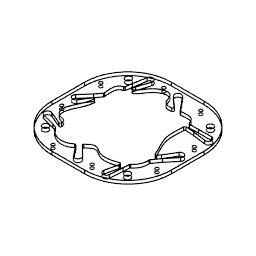
MidPlateShell_v29 (Autodesk Fusion 360 design; units mm, degrees)
Autodesk Fusion 360 part; units mm, degrees
(part 1 of 2)
sketch "Sketch1" plane through (0, 0, 0) normal (0, 0, 1) x (1, 0, 0)
  line L0 (-33.4, -17.4) -> (-33.4, 33.4) construction
  line L1 (-33.4, 33.4) -> (-27.4, 33.4) construction
  line L2 (-33.4, -17.4) -> (-36.4, -17.4)
  line L3 (-36.4, -17.4) -> (-36.4, -27.4)
  line L4 (-36.4, -27.4) -> (-33.4, -27.4)
  line L5 (-33.4, -27.4) -> (-33.4, -17.4)
  line L6 (-27.4, 33.4) -> (-17.4, 33.4)
  line L7 (-17.4, 33.4) -> (-17.4, 36.4)
  line L8 (-17.4, 36.4) -> (-27.4, 36.4)
  line L9 (-27.4, 36.4) -> (-27.4, 33.4)
  line L10 (-17.4, 33.4) -> (33.4, 33.4) construction
  line L11 (33.4, 33.4) -> (33.4, 27.4) construction
  line L12 (33.4, 27.4) -> (36.4, 27.4)
  line L13 (36.4, 27.4) -> (36.4, 17.4)
  line L14 (36.4, 17.4) -> (33.4, 17.4)
  line L15 (33.4, 17.4) -> (33.4, 27.4)
  line L16 (33.4, 17.4) -> (33.4, -33.4) construction
  line L17 (33.4, -33.4) -> (27.4, -33.4) construction
  line L18 (27.4, -33.4) -> (17.4, -33.4)
  line L19 (17.4, -33.4) -> (17.4, -36.4)
  line L20 (17.4, -36.4) -> (27.4, -36.4)
  line L21 (27.4, -36.4) -> (27.4, -33.4)
  line L22 (17.4, -33.4) -> (-33.4, -33.4) construction
  line L23 (-33.4, -33.4) -> (-33.4, -27.4) construction
  line L24 (33.4, 33.4) -> (-33.4, -33.4) construction
  line L25 (33.4, -33.4) -> (-33.4, 33.4) construction
  line L26 (55, -55) -> (-55, -55)
  line L27 (-55, -55) -> (-55, 55)
  line L28 (-55, 55) -> (55, 55)
  line L29 (55, 55) -> (55, -55)
  line L30 (55, -55) -> (-55, 55) construction
  line L31 (-55, -55) -> (55, 55) construction
  line L32 (-34.9, -17.4) -> (-34.9, -7.75) construction
  line L33 (-34.9, -7.75) -> (-38.15, -7.75) construction
  circle A0 centre (-38.15, -7.75) radius 1.25
  line L34 (-34.9, -27.4) -> (-34.9, -38.15) construction
  line L35 (-34.9, -38.15) -> (-37.75, -38.15) construction
  circle A1 centre (-37.75, -38.15) radius 1.25
  circle A2 centre (38.15, -37.75) radius 1.25
  circle A3 centre (7.75, -38.15) radius 1.25
  circle A4 centre (37.75, 38.15) radius 1.25
  circle A5 centre (38.15, 7.75) radius 1.25
  circle A6 centre (-38.15, 37.75) radius 1.25
  circle A7 centre (-7.75, 38.15) radius 1.25
  constraint vertical L0
  constraint perpendicular L0 L1
  constraint horizontal L2
  constraint vertical L3
  constraint horizontal L4
  constraint vertical L5
  constraint horizontal L6
  constraint vertical L7
  constraint horizontal L8
  constraint vertical L9
  constraint perpendicular L7 L10
  constraint perpendicular L10 L11
  constraint horizontal L12
  constraint vertical L13
  constraint horizontal L14
  constraint vertical L15
  constraint perpendicular L14 L16
  constraint perpendicular L16 L17
  constraint horizontal L18
  constraint vertical L19
  constraint horizontal L20
  constraint vertical L21
  constraint perpendicular L19 L22
  constraint coincident origin L24
  constraint coincident origin L25
  constraint horizontal L26
  constraint perpendicular L26 L27
  constraint parallel L26 L28
  constraint parallel L27 L29
  constraint coincident L30 origin
  constraint coincident L31 origin
  constraint midpoint L2 L32.start
  constraint perpendicular L2 L32
  constraint perpendicular L32 L33
  constraint coincident L33.end A0.centre
  constraint midpoint L4 L34.start
  constraint perpendicular L4 L34
  constraint perpendicular L34 L35
  constraint coincident L35.end A1.centre
  measures "d1" distance of L0.start L0.end
  measures "d2" distance of L0.end L1.end
  measures "d3" distance of L0.start L2.end
  measures "d4" distance of L0.start L4.end
  measures "d5" distance of L1.end L6.end
  measures "d6" distance of L1.end L8.end
  measures "d7" distance of L6.end L10.end
  measures "d8" distance of L10.end L11.end
  measures "d9" distance of L11.end L12.end
  measures "d10" distance of L11.end L14.end
  measures "d11" distance of L14.end L16.end
  measures "d12" distance of L16.end L17.end
  measures "d13" distance of L17.end L18.end
  measures "d14" distance of L17.end L20.end
  measures "d15" distance of L18.end L22.end
  measures "d16" distance of L27.end L28.end
  measures "d17" distance of L26.end L27.end
  measures "d22" distance of L32.start L32.end
  measures "d23" distance of L32.end L33.end
  measures "d24" diameter of A0
  measures "d25" distance of L34.start L34.end
  measures "d26" distance of L34.end L35.end
  measures "d27" diameter of A1
extrude "Extrude1" add sketch "Sketch1" along normal blind 3 contours L2 L3 L4 L5 | L6 L7 L8 L9 | L12 L13 L14 L15 | L18 L19 L20 L21 | L26 L27 L28 L29 | A0 | A1 | A2 | A3 | A4 | A5 | A6 | A7 picked at (-35.4, -24.066667) picked at (-24.066667, 35.4) picked at (34.4, 24.066667) picked at (20.733333, -34.4) picked at (-5.8, 11.133333) picked at (-38.302225, -8.262066) picked at (-38.630134, -38.247182) picked at (37.269866, -37.847182) picked at (7.417812, -38.501562) picked at (36.869866, 38.052818) picked at (37.997775, 7.237934) picked at (-39.030134, 37.652818) picked at (-8.082188, 37.798438)
fillet "Fillet1" radius 40 4 edges at (-55, 55, 1.5) (55, 55, 1.5) (55, -55, 1.5) (-55, -55, 1.5)
other "Sketch1 (1)"
sketch "sketch 2514" plane through (0, 0, 0) normal (0, 0, 1) x (1, 0, 0)
  line L0 (55, -55) -> (-55, -55)
  line L1 (-55, -55) -> (-55, 55)
  line L2 (-55, 55) -> (55, 55)
  line L3 (55, 55) -> (55, -55)
  circle A0 centre (-27, 47.000001) radius 3
  circle A1 centre (-1, 47.000001) radius 3
  circle A2 centre (-47.000001, -1) radius 3
  circle A3 centre (-47.000001, -27) radius 3
  circle A4 centre (3.826834, 9.238795) radius 2.1
  line L4 (3.826834, 9.238795) -> (0, 0) construction
  circle A5 centre (-3.826834, 9.238795) radius 2.1
  circle A6 centre (-9.238795, 3.826834) radius 2.1
  circle A7 centre (-9.238795, -3.826834) radius 2.1
  circle A8 centre (-3.826834, -9.238795) radius 2.1
  circle A9 centre (3.826834, -9.238795) radius 2.1
  circle A10 centre (9.238795, -3.826834) radius 2.1
  circle A11 centre (9.238795, 3.826834) radius 2.1
  circle A12 centre (-47.000001, -27) radius 3
  circle A13 centre (-47.000001, -1) radius 3
  circle A14 centre (27, -47.000001) radius 3
  circle A15 centre (1, -47.000001) radius 3
  circle A16 centre (47.000001, 27) radius 3
  circle A17 centre (47.000001, 1) radius 3
  line L5 (3.826834, 9.238795) -> (-7.355951, 51.448425) construction
  line L6 (-3.826709, 9.238713) -> (-39.148117, 32.338774) construction
  line L7 (-9.224092, 3.83023) -> (-38.107832, -2.83954) construction
  line L8 (-9.238692, -3.826753) -> (-45.731263, -32.409069) construction
  line L9 (-3.841818, -9.257167) -> (-24.537186, -34.631992) construction
  line L10 (3.826834, -9.238795) -> (20.713135, -35.705512) construction
  line L11 (9.238772, -3.82683) -> (32.789694, -8.144866) construction
  line L12 (9.238795, 3.826834) -> (22.419532, 22.467528) construction
  line L13 (0, 0) -> (0, 3) construction
  line L14 (-38.107832, -2.83954) -> (1, -47.000001) construction
  line L15 (32.789694, -8.144866) -> (27, -47.000001) construction
  line L16 (20.713135, -35.705512) -> (47.000001, 1) construction
  line L17 (-39.148117, 32.338774) -> (47.000001, 27) construction
  line L18 (22.419532, 22.467528) -> (-1, 47.000001) construction
  line L19 (-45.731263, -32.409069) -> (-27, 47.000001) construction
  line L20 (-24.537186, -34.631992) -> (-47.000001, -27) construction
  line L21 (-7.355951, 51.448425) -> (-47.000001, -1) construction
  circle A18 centre (-26.92648, -6.415459) radius 6 construction
  circle A19 centre (-26.552885, -27.610279) radius 6 construction
  circle A20 centre (21, -25) radius 6 construction
  circle A21 centre (26, -13) radius 6 construction
  circle A22 centre (14.668303, 21.897871) radius 6 construction
  circle A23 centre (-10, 38.000001) radius 6 construction
  circle A24 centre (-16.884287, 24.947529) radius 6 construction
  circle A25 centre (-35.96441, -17.137991) radius 6 construction
  line L22 (-1.27632, 20.300794) -> (2.783612, 21.37641)
  line L23 (-1.27632, 20.300794) -> (1.796868, 8.700987) construction
  line L24 (2.783612, 21.37641) -> (5.8568, 9.776603) construction
  line L25 (-15.019188, 14.049327) -> (-12.720372, 17.564358)
  line L26 (-20.458615, -0.919284) -> (-21.403603, 3.173026)
  line L27 (-19.980867, -9.572955) -> (-17.391085, -12.879468)
  line L28 (-13.038601, -17.210832) -> (-9.783844, -19.865367)
  line L29 (8.510904, -20.484661) -> (12.051623, -18.22561)
  line L30 (21.420761, -3.925379) -> (20.663322, -8.056515)
  line L31 (14.452267, 14.837271) -> (17.881573, 12.412427)
  line L32 (-12.720372, 17.564358) -> (-2.677426, 10.996311) construction
  line L33 (-15.019188, 14.049327) -> (-4.976243, 7.48128) construction
  line L34 (-21.403603, 3.173026) -> (-9.711289, 5.872989) construction
  line L35 (-20.458615, -0.919284) -> (-8.766302, 1.780679) construction
  line L36 (-19.980867, -9.572955) -> (-10.533686, -2.173578) construction
  line L37 (-17.391085, -12.879468) -> (-7.943904, -5.480091) construction
  line L38 (-9.783844, -19.865367) -> (-2.199456, -10.566063) construction
  line L39 (-13.038601, -17.210832) -> (-5.454213, -7.911527) construction
  line L40 (12.051623, -18.22561) -> (5.597194, -8.10927) construction
  line L41 (8.510904, -20.484661) -> (2.056475, -10.368321) construction
  line L42 (20.663322, -8.056515) -> (8.860076, -5.892402) construction
  line L43 (21.420761, -3.925379) -> (9.617515, -1.761266) construction
  line L44 (14.452267, 14.837271) -> (7.524143, 5.039256) construction
  line L45 (17.881573, 12.412427) -> (10.953448, 2.614413) construction
  line L46 (26.691493, -34.821543) -> (30.845628, -35.440539)
  line L47 (-8.527907, -39.408625) -> (-5.383635, -36.624105)
  line L48 (-34.962331, -28.872033) -> (-36.313471, -32.848768)
  line L49 (-41.439374, 9.839254) -> (-38.088834, 7.30669)
  line L50 (-31.798898, 35.802654) -> (-27.711083, 34.838407)
  line L51 (5.767132, 36.870049) -> (8.805091, 39.770188)
  line L52 (35.15287, 29.83822) -> (34.893086, 25.646262)
  line L53 (38.305738, -7.533451) -> (41.720395, -9.978878)
  line L54 (30.845628, -35.440539) -> (29.992153, -47.216854)
  line L55 (26.691493, -34.821543) -> (24.074611, -46.335098)
  line L56 (-5.383635, -36.624105) -> (3.089335, -44.84717)
  line L57 (-8.527907, -39.408625) -> (-1.389663, -48.813702)
  line L58 (-34.962331, -28.872033) -> (-45.823197, -24.240447)
  line L59 (-36.313471, -32.848768) -> (-47.747888, -29.90528)
  line L60 (-41.439374, 9.839254) -> (-49.249836, 0.9845)
  line L61 (-38.088834, 7.30669) -> (-44.477012, -2.623123)
  line L62 (-27.711083, 34.838407) -> (-24.140467, 46.09277)
  line L63 (-31.798898, 35.802654) -> (-29.963534, 47.466334)
  line L64 (8.805091, 39.770188) -> (1.320176, 48.901784)
  line L65 (5.767132, 36.870049) -> (-3.007378, 44.770554)
  line L66 (35.15287, 29.83822) -> (46.958966, 29.99972)
  line L67 (34.893086, 25.646262) -> (46.588905, 24.0283)
  line L68 (41.720395, -9.978878) -> (49.300203, -0.925894)
  line L69 (38.305738, -7.533451) -> (44.436043, 2.557602)
  circle A26 centre (-10, 38.000001) radius 1.5
  circle A27 centre (-17, 25) radius 1.5
  circle A28 centre (14.668303, 21.897871) radius 1.5
  circle A29 centre (-26.92648, -6.415459) radius 1.5
  circle A30 centre (-36.000001, -17) radius 1.5
  circle A31 centre (-26.552885, -27.610279) radius 1.5
  circle A32 centre (21, -25) radius 1.5
  circle A33 centre (26, -13) radius 1.5
  line L70 (-13.86978, 15.806842) -> (-3.826834, 9.238795) construction
  line L71 (0.753646, 20.838602) -> (3.826834, 9.238795) construction
  line L72 (9.238795, 3.826834) -> (16.16692, 13.624849) construction
  line L73 (9.238795, -3.826834) -> (21.042041, -5.990947) construction
  line L74 (3.826834, -9.238795) -> (10.281264, -19.355135) construction
  line L75 (-3.841818, -9.257167) -> (-11.411222, -18.5381) construction
  line L76 (-9.238795, -3.826834) -> (-18.685976, -11.226211) construction
  line L77 (-9.224092, 3.83023) -> (-20.931109, 1.126871) construction
  line L78 (-11.034179, 9.172896) -> (-6.655482, 15.868194) construction
  line L79 (-15.977588, 6.375988) -> (-14.177613, -1.418888) construction
  line L80 (-16.428845, -4.377463) -> (-11.495926, -10.675583) construction
  line L81 (-10.726288, -11.369504) -> (-4.526752, -16.425763) construction
  line L82 (3.681936, -16.448442) -> (10.426163, -12.145489) construction
  line L83 (15.861789, -0.974475) -> (14.419048, -8.843306) construction
  line L84 (9.436853, 11.035216) -> (15.968862, 6.416467) construction
  line L85 (-1.576362, 14.014302) -> (6.156842, 16.063095) construction
  line L86 (-7.91085, 16.689199) -> (-5.400113, 15.047188)
  line L87 (5.772694, 17.513071) -> (6.540991, 14.613119)
  line L88 (-1.960511, 15.464278) -> (-1.192214, 12.564327)
  line L89 (-12.289548, 9.993902) -> (-9.778811, 8.35189)
  line L90 (-17.439128, 6.038493) -> (-14.516049, 6.713484)
  line L91 (-15.639152, -1.756383) -> (-12.716074, -1.081392)
  line L92 (-17.609742, -5.302385) -> (-15.247947, -3.452541)
  line L93 (-12.676824, -11.600505) -> (-10.315029, -9.750661)
  line L94 (-11.674336, -12.531917) -> (-9.778239, -10.207091)
  line L95 (-5.4748, -17.588176) -> (-3.578703, -15.26335)
  line L96 (2.875132, -15.183899) -> (4.488739, -17.712984)
  line L97 (9.619359, -10.880946) -> (11.232966, -13.410031)
  line L98 (12.943642, -8.572792) -> (15.894453, -9.11382)
  line L99 (14.386383, -0.703961) -> (17.337195, -1.244989)
  line L100 (16.834878, 7.641219) -> (15.102847, 5.191715)
  line L101 (10.302868, 12.259968) -> (8.570837, 9.810465)
  line L102 (5.772694, 17.513071) -> (3.936058, 17.026482)
  line L103 (6.540991, 14.613119) -> (4.704355, 14.126531)
  line L104 (-1.960511, 15.464278) -> (-0.123875, 15.950866)
  line L105 (-1.192214, 12.564327) -> (0.644422, 13.050915)
  line L106 (-7.91085, 16.689199) -> (-8.881368, 15.053664)
  line L107 (-5.400113, 15.047188) -> (-6.440054, 13.457055)
  line L108 (-12.289548, 9.993902) -> (-11.249607, 11.584035)
  line L109 (-9.778811, 8.35189) -> (-8.73887, 9.942024)
  line L110 (-17.439128, 6.038493) -> (-17.011633, 4.18721)
  line L111 (-14.516049, 6.713484) -> (-14.088555, 4.862201)
  line L112 (-12.716074, -1.081392) -> (-13.143568, 0.769891)
  line L113 (-15.639152, -1.756383) -> (-16.066646, 0.0949)
  line L114 (-15.247947, -3.452541) -> (-14.076379, -4.948344)
  line L115 (-17.609742, -5.302385) -> (-16.438174, -6.798188)
  line L116 (-10.315029, -9.750661) -> (-11.486597, -8.254857)
  line L117 (-12.676824, -11.600505) -> (-13.848392, -10.104702)
  line L118 (-9.778239, -10.207091) -> (-8.30585, -11.407952)
  line L119 (-11.674336, -12.531917) -> (-10.201947, -13.732778)
  line L120 (-3.578703, -15.26335) -> (-5.051093, -14.062488)
  line L121 (-5.4748, -17.588176) -> (-6.94719, -16.387314)
  line L122 (2.875132, -15.183899) -> (4.476886, -14.161948)
  line L123 (4.488739, -17.712984) -> (6.090493, -16.691033)
  line L124 (11.232966, -13.410031) -> (9.631212, -14.431983)
  line L125 (9.619359, -10.880946) -> (8.017605, -11.902898)
  line L126 (15.894453, -9.11382) -> (16.237104, -7.244973)
  line L127 (12.943642, -8.572792) -> (13.286293, -6.703945)
  line L128 (17.337195, -1.244989) -> (16.994544, -3.113837)
  line L129 (14.386383, -0.703961) -> (14.043732, -2.572808)
  line L130 (16.834878, 7.641219) -> (15.283526, 8.738172)
  line L131 (15.102847, 5.191715) -> (13.551495, 6.288668)
  line L132 (8.570837, 9.810465) -> (10.12219, 8.713512)
  line L133 (10.302868, 12.259968) -> (11.854221, 11.163015)
  line L134 (-6.955771, -38.016365) -> (1, -47.000001) construction
  line L135 (27, -47.000001) -> (28.76856, -35.131041) construction
  line L136 (47.000001, 1) -> (40.013067, -8.756165) construction
  line L137 (47.000001, 27) -> (35.022978, 27.742241) construction
  line L138 (-1, 47.000001) -> (7.286111, 38.320118) construction
  line L139 (-27, 47.000001) -> (-29.754991, 35.32053) construction
  line L140 (-47.000001, -1) -> (-39.764104, 8.572972) construction
  line L141 (-47.000001, -27) -> (-35.637901, -30.8604) construction
  line L142 (-6.721067, -45.823087) -> (0.765296, -39.193278) construction
  line L143 (22.938881, -40.328621) -> (32.82968, -41.802421) construction
  line L144 (39.441465, -0.96686) -> (47.571602, -6.789305) construction
  line L145 (41.320756, 32.361547) -> (40.702222, 22.380694) construction
  line L146 (-0.473562, 39.207513) -> (6.759673, 46.112606) construction
  line L147 (-33.243942, 42.308178) -> (-23.51105, 40.012353) construction
  line L148 (-47.370791, 6.801443) -> (-39.393314, 0.771529) construction
  line L149 (-39.710451, -24.195992) -> (-42.927451, -33.664409) construction
  line L150 (-7.715538, -44.700133) -> (-5.726596, -46.946042)
  line L151 (-0.229175, -38.070324) -> (1.759767, -40.316233)
  line L152 (23.159951, -38.845001) -> (22.717811, -41.812241)
  line L153 (33.05075, -40.318801) -> (32.60861, -43.286041)
  line L154 (38.568098, -2.18638) -> (40.314832, 0.252661)
  line L155 (46.698236, -8.008826) -> (48.444969, -5.569784)
  line L156 (39.205094, 22.473474) -> (42.19935, 22.287914)
  line L157 (39.823628, 32.454327) -> (42.817884, 32.268767)
  line L158 (-1.509326, 40.292498) -> (0.562202, 38.122528)
  line L159 (5.723909, 47.197591) -> (7.795437, 45.02762)
  line L160 (-32.899568, 43.768112) -> (-33.588315, 40.848244)
  line L161 (-23.855423, 38.552419) -> (-23.166676, 41.472287)
  line L162 (-48.275278, 5.604822) -> (-46.466304, 7.998065)
  line L163 (-40.297801, -0.425092) -> (-38.488827, 1.968151)
  line L164 (-41.130713, -23.713442) -> (-38.290188, -24.678542)
  line L165 (-44.347713, -33.181859) -> (-41.507188, -34.146959)
  line L166 (-7.715538, -44.700133) -> (-5.799569, -43.003379)
  line L167 (-5.726596, -46.946042) -> (-3.980676, -45.399882)
  line L168 (-0.229175, -38.070324) -> (-2.145145, -39.767078)
  line L169 (1.759767, -40.316233) -> (0.013848, -41.862393)
  line L170 (23.159951, -38.845001) -> (25.691283, -39.222188)
  line L171 (22.717811, -41.812241) -> (25.024477, -42.155951)
  line L172 (33.05075, -40.318801) -> (30.519418, -39.941614)
  line L173 (32.60861, -43.286041) -> (30.301944, -42.942331)
  line L174 (40.314832, 0.252661) -> (42.210888, -1.105211)
  line L175 (38.568098, -2.18638) -> (40.648828, -3.676507)
  line L176 (48.444969, -5.569784) -> (46.548913, -4.211913)
  line L177 (46.698236, -8.008826) -> (44.617506, -6.518699)
  line L178 (39.823628, 32.454327) -> (39.665328, 29.899947)
  line L179 (42.817884, 32.268767) -> (42.673634, 29.941099)
  line L180 (42.19935, 22.287914) -> (42.343601, 24.615582)
  line L181 (39.205094, 22.473474) -> (39.363395, 25.027854)
  line L182 (-1.509326, 40.292498) -> (0.177561, 41.902858)
  line L183 (0.562202, 38.122528) -> (2.413389, 39.889734)
  line L184 (7.795437, 45.02762) -> (5.94425, 43.260414)
  line L185 (5.723909, 47.197591) -> (4.037023, 45.587231)
  line L186 (-32.899568, 43.768112) -> (-30.629728, 43.232695)
  line L187 (-33.588315, 40.848244) -> (-31.097396, 40.260678)
  line L188 (-23.166676, 41.472287) -> (-25.436516, 42.007704)
  line L189 (-23.855423, 38.552419) -> (-26.346343, 39.139985)
  line L190 (-46.466304, 7.998065) -> (-44.424644, 6.454841)
  line L191 (-48.275278, 5.604822) -> (-46.414824, 4.198565)
  line L192 (-38.488827, 1.968151) -> (-40.530486, 3.511374)
  line L193 (-40.297801, -0.425092) -> (-42.158255, 0.981164)
  line L194 (-38.290188, -24.678542) -> (-39.113509, -27.101775)
  line L195 (-41.130713, -23.713442) -> (-41.880961, -25.921603)
  line L196 (-41.507188, -34.146959) -> (-40.683868, -31.723724)
  line L197 (-44.347713, -33.181859) -> (-43.597465, -30.973695)
  line L198 (1, -47.000001) -> (27, -47.000001) construction
  line L199 (-47.000001, -1) -> (-47.000001, -27) construction
  line L200 (47.000001, 1) -> (47.000001, 27) construction
  line L201 (-1, 47.000001) -> (-27, 47.000001) construction
  circle A34 centre (14, -47.000001) radius 1.5
  circle A35 centre (-47.000001, -14) radius 1.5
  circle A36 centre (47.000001, 14) radius 1.5
  circle A37 centre (-14, 47.000001) radius 1.5
  circle A38 centre (0, 0) radius 6
  line L202 (-15.511792, 13.296106) -> (-12.227769, 18.317579)
  line L203 (-21.6061, 4.049949) -> (-20.256118, -1.796207)
  line L204 (-20.53582, -8.864416) -> (-16.836131, -13.588007)
  line L205 (-13.736048, -16.642003) -> (-9.086396, -20.434197)
  line L206 (7.752179, -20.968743) -> (12.810349, -17.741528)
  line L207 (20.501013, -8.941758) -> (21.583069, -3.040135)
  line L208 (13.717416, 15.35688) -> (18.616424, 11.892818)
  line L209 (-2.146306, 20.070305) -> (3.653597, 21.606899)
  line L210 (1.796868, 8.700987) -> (-2.146306, 20.070305)
  line L211 (3.653597, 21.606899) -> (5.8568, 9.776603)
  line L212 (13.717416, 15.35688) -> (7.43879, 4.90849)
  line L213 (18.616424, 11.892818) -> (10.953448, 2.614413)
  line L214 (21.583069, -3.040135) -> (9.617515, -1.761266)
  line L215 (20.501013, -8.941758) -> (8.860076, -5.892402)
  line L216 (12.810349, -17.741528) -> (5.597194, -8.10927)
  line L217 (7.752179, -20.968743) -> (2.056475, -10.368321)
  line L218 (-13.736048, -16.642003) -> (-5.454213, -7.911527)
  line L219 (-9.086396, -20.434197) -> (-2.199456, -10.566063)
  line L220 (-20.53582, -8.864416) -> (-10.533686, -2.173578)
  line L221 (-16.836131, -13.588007) -> (-7.943904, -5.480091)
  line L222 (-21.6061, 4.049949) -> (-9.711289, 5.872989)
  line L223 (-20.256118, -1.796207) -> (-8.615561, 1.821447)
  line L224 (-15.511792, 13.296106) -> (-4.842466, 7.400728)
  line L225 (-12.227769, 18.317579) -> (-2.677426, 10.996311)
  point P0 (0.753646, 20.838602)
  point P1 (-13.86978, 15.806842)
  point P2 (-20.931109, 1.126871)
  point P3 (-18.685976, -11.226211)
  point P4 (-11.411222, -18.5381)
  point P5 (10.281264, -19.355135)
  point P6 (21.042041, -5.990947)
  point P7 (16.16692, 13.624849)
  point P8 (28.76856, -35.131041)
  point P9 (-6.955771, -38.016365)
  point P10 (-35.637901, -30.8604)
  point P11 (-39.764104, 8.572972)
  point P12 (-29.754991, 35.32053)
  point P13 (7.286111, 38.320118)
  point P14 (35.022978, 27.742241)
  point P15 (40.013067, -8.756165)
  point P16 (-8.84483, 12.520545)
  point P17 (-15.077601, 2.47855)
  point P18 (-13.962386, -7.526523)
  point P19 (-7.62652, -13.897634)
  point P20 (7.054049, -14.296965)
  point P21 (15.140418, -4.908891)
  point P22 (12.702858, 8.725842)
  point P23 (2.29024, 15.038699)
  point P24 (-2.977885, -42.508183)
  point P25 (27.88428, -41.065521)
  point P26 (43.506534, -3.878082)
  point P27 (41.011489, 27.371121)
  point P28 (3.143056, 42.660059)
  point P29 (-28.377496, 41.160266)
  point P30 (-43.382052, 3.786486)
  point P31 (-41.318951, -28.9302)
extrude "Extrude6" cut sketch "sketch 2514" along normal blind 9 contours A0 | A0 L50 L62 L63 | A1 | A1 L51 L64 L65 | A2 A13 | A2 A13 L49 L60 L61 | A3 A12 | A3 A12 L48 L58 L59 | A14 | A14 L46 L54 L55 | A15 | A15 L47 L56 L57 | A16 | A16 L52 L66 L67 | A17 | A17 L53 L68 L69 picked at (-26.071156, 46.419358) picked at (-28.377496, 41.160266) picked at (-1.17985, 46.053439) picked at (3.101996, 42.622978) picked at (-47.821295, -1.752419) picked at (-43.327834, 3.742446) picked at (-46.145825, -27.653089) picked at (-41.304854, -28.885262) picked at (28.422001, -46.164814) picked at (27.848413, -41.060838) picked at (0.277691, -48.202794) picked at (-2.977885, -42.508183) picked at (47.846051, 26.373339) picked at (41.011489, 27.371121) picked at (47.712465, 0.007779) picked at (43.506534, -3.878082)
sketch "Sketch3" plane through (0, 0, 0) normal (0, 0, -1) x (1, 0, 0)
  arc A0 (-15, 55) -> (-55, 15) centre (-15, 15) ccw
  line L0 (-55, 15) -> (-55, -15)
  arc A1 (-55, -15) -> (-15, -55) centre (-15, -15) ccw
  line L1 (-15, -55) -> (15, -55)
  arc A2 (15, -55) -> (55, -15) centre (15, -15) ccw
  line L2 (55, -15) -> (55, 15)
  arc A3 (55, 15) -> (15, 55) centre (15, 15) ccw
  line L3 (15, 55) -> (-15, 55)
  line L4 (30.845628, 35.440539) -> (26.691493, 34.821543)
  line L5 (26.691493, 34.821543) -> (24.074611, 46.335098)
  arc A4 (29.992153, 47.216854) -> (24.074611, 46.335098) centre (27, 47.000001) ccw
  line L6 (29.992153, 47.216854) -> (30.845628, 35.440539)
  arc A5 (-3.007378, -44.770554) -> (1.320176, -48.901784) centre (-1, -47.000001) ccw
  line L7 (-3.007378, -44.770554) -> (5.767132, -36.870049)
  line L8 (5.767132, -36.870049) -> (8.805091, -39.770188)
  line L9 (8.805091, -39.770188) -> (1.320176, -48.901784)
  line L10 (-36.313471, 32.848768) -> (-34.962331, 28.872033)
  line L11 (-34.962331, 28.872033) -> (-45.823197, 24.240447)
  arc A6 (-47.747889, 29.905282) -> (-45.823197, 24.240447) centre (-47.000001, 27) ccw
  line L12 (-47.747889, 29.905282) -> (-36.313471, 32.848768)
  arc A7 (46.958966, -29.99972) -> (46.588905, -24.0283) centre (47.000001, -27) ccw
  line L13 (46.958966, -29.99972) -> (35.15287, -29.83822)
  line L14 (35.15287, -29.83822) -> (34.893086, -25.646262)
  line L15 (34.893086, -25.646262) -> (46.588905, -24.0283)
  line L16 (-5.383635, 36.624105) -> (-8.527907, 39.408625)
  line L17 (-8.527907, 39.408625) -> (-1.389663, 48.813702)
  arc A8 (3.089335, 44.84717) -> (-1.389663, 48.813702) centre (1, 47.000001) ccw
  line L18 (3.089335, 44.84717) -> (-5.383635, 36.624105)
  arc A9 (-29.963534, -47.466334) -> (-24.140467, -46.09277) centre (-27, -47.000001) ccw
  line L19 (-29.963534, -47.466334) -> (-31.798898, -35.802654)
  line L20 (-31.798898, -35.802654) -> (-27.711083, -34.838407)
  line L21 (-27.711083, -34.838407) -> (-24.140467, -46.09277)
  line L22 (-38.088834, -7.30669) -> (-41.439374, -9.839254)
  line L23 (-41.439374, -9.839254) -> (-49.249836, -0.9845)
  arc A10 (-44.477012, 2.623123) -> (-49.249836, -0.9845) centre (-47.000001, 1) ccw
  line L24 (-44.477012, 2.623123) -> (-38.088834, -7.30669)
  arc A11 (44.436043, -2.557602) -> (49.300203, 0.925894) centre (47.000001, -1) ccw
  line L25 (44.436043, -2.557602) -> (38.305738, 7.533451)
  line L26 (38.305738, 7.533451) -> (41.720395, 9.978878)
  line L27 (41.720395, 9.978878) -> (49.300203, 0.925894)
  spline S0 degree 5 poles (6, 33) (5.616128, 32.772866) (4.858533, 32.312893) (3.745533, 31.631813) (2.284945, 30.869856) (0.451972, 30.499595) (-1.43328, 30.97008) (-3.428192, 32.345509) (-5.608083, 34.431048) (-8.044412, 36.876587) (-10.78785, 39.251814) (-13.848701, 41.134247) (-17.18009, 42.187697) (-20.655936, 42.254534) (-24.06337, 41.412642) (-27.158, 39.883449) (-29.708435, 37.963846) (-31.548468, 35.943843) (-32.618058, 34.04182) (-33.028847, 32.303849) (-33.042381, 30.628698) (-32.961424, 28.914986) (-33.041736, 27.183431) (-33.402956, 25.689575) (-34.08315, 24.706116) (-35.095124, 24.28536) (-36.458005, 24.121881) (-38.135285, 23.810799) (-39.967248, 23.090006) (-41.704841, 21.873503) (-43.090697, 20.179057) (-43.923497, 18.091574) (-44.1323, 15.71051) (-43.751109, 13.13653) (-42.890611, 10.456347) (-41.711167, 7.729261) (-40.394767, 4.970947) (-39.119097, 2.144358) (-38.041891, -0.812208) (-37.283996, -3.961635) (-36.91295, -7.342775) (-36.926225, -10.945892) (-37.234751, -14.687973) (-37.645802, -18.387573) (-37.914865, -21.815217) (-37.796648, -24.743101) (-37.098701, -26.997141) (-35.728731, -28.503301) (-33.757232, -29.34785) (-31.433833, -29.79556) (-29.070042, -30.186421) (-26.945382, -30.853784) (-25.205449, -32.034771) (-23.760214, -33.781991) (-22.377064, -36.001435) (-20.777292, -38.493403) (-18.733074, -40.992199) (-16.160001, -43.20627) (-13.223019, -44.858225) (-10.238953, -45.720625) (-7.564781, -45.650278) (-5.487372, -44.625275) (-4.121085, -42.77605) (-3.27943, -40.432058) (-2.573014, -38.035979) (-1.554615, -36.028725) (0.162958, -34.754174) (2.75224, -34.333045) (6.123234, -34.630938) (10.019984, -35.355222) (14.081948, -36.12046) (17.919474, -36.526428) (21.183306, -36.230845) (23.636437, -35.024107) (25.225651, -32.904025) (26.038332, -30.017752) (26.259039, -26.603889) (26.125194, -22.932557) (25.885595, -19.251037) (25.751825, -15.715548) (25.8753, -12.372768) (26.353104, -9.197249) (27.226276, -6.114073) (28.481055, -3.027599) (30.048992, 0.152694) (31.807108, 3.484454) (33.579128, 6.967394) (35.159985, 10.557354) (36.339284, 14.178551) (36.924834, 17.736374) (36.766884, 21.130182) (35.78041, 24.265512) (33.972284, 27.067933) (31.453968, 29.491912) (28.404926, 31.512762) (25.043906, 33.121234) (21.597622, 34.317361) (18.269518, 35.10399) (15.210937, 35.481959) (12.484828, 35.440643) (10.079867, 34.979402) (8.366092, 34.305453) (7.161763, 33.675702) (6.383872, 33.227135) (6, 33) knots 0 0 0 0 0 0 0.01 0.02 0.03 0.04 0.05 0.06 0.07 0.08 0.09 0.1 0.11 0.12 0.13 0.14 0.15 0.16 0.17 0.18 0.19 0.2 0.21 0.22 0.23 0.24 0.25 0.26 0.27 0.28 0.29 0.3 0.31 0.32 0.33 0.34 0.35 0.36 0.37 0.38 0.39 0.4 0.41 0.42 0.43 0.44 0.45 0.46 0.47 0.48 0.49 0.5 0.51 0.52 0.53 0.54 0.55 0.56 0.57 0.58 0.59 0.6 0.61 0.62 0.63 0.64 0.65 0.66 0.67 0.68 0.69 0.7 0.71 0.72 0.73 0.74 0.75 0.76 0.77 0.78 0.79 0.8 0.81 0.82 0.83 0.84 0.85 0.86 0.87 0.88 0.89 0.9 0.91 0.92 0.93 0.94 0.95 0.96 0.97 0.98 0.99 1 1 1 1 1 1
  line L28 (-31.798898, -35.802654) -> (-32.790801, -29.49158)
  line L29 (-27.711083, -34.838407) -> (-28.770264, -30.348131)
  line L30 (5.767132, -36.870049) -> (7.610633, -34.938941)
  line L31 (8.805091, -39.770188) -> (12.116839, -35.729853)
  line L32 (34.893086, -25.646262) -> (26.175138, -26.186531)
  line L33 (35.15287, -29.83822) -> (25.919241, -29.71354)
  line L34 (41.720395, 9.978878) -> (36.68528, 17.009632)
  line L35 (38.305738, 7.533451) -> (35.421022, 11.561507)
  line L36 (26.691493, 34.821543) -> (27.102043, 32.066301)
  line L37 (30.845628, 35.440539) -> (31.281435, 29.423422)
  line L38 (-5.383635, 36.624105) -> (-6.519453, 35.341542)
  line L39 (-8.527907, 39.408625) -> (-9.625144, 38.169628)
  line L40 (-36.313471, 32.848768) -> (-32.415986, 34.172982)
  line L41 (-34.962331, 28.872033) -> (-33.002634, 29.537862)
  line L42 (-38.088834, -7.30669) -> (-36.964405, -8.794291)
  line L43 (-41.439374, -9.839254) -> (-37.317874, -15.291931)
  point P0 (-1, 31)
  point P1 (-16.538047, 41.812241)
  point P2 (-32, 35.000001)
  point P3 (-33, 29)
  point P4 (-34.000001, 25)
  point P5 (-37.000001, 24)
  point P6 (-43.000001, 20)
  point P7 (-41.880961, 8.179159)
  point P8 (-37.000001, -11)
  point P9 (-36.000001, -28)
  point P10 (-27, -31)
  point P11 (-18.417002, -41.106785)
  point P12 (-5.390348, -44.179517)
  point P13 (-0.456665, -35.394099)
  point P14 (21, -36.000001)
  point P15 (26, -21)
  point P16 (30, 0)
  point P17 (35.88208, 23.473736)
  point P18 (17.657226, 35.117392)
  constraint perpendicular L20 L29
  constraint perpendicular L8 L30
  constraint parallel L9 L31
  constraint perpendicular L14 L32
  constraint perpendicular L26 L34
  constraint perpendicular L26 L35
  constraint perpendicular L4 L36
  constraint perpendicular L16 L38
  constraint perpendicular L16 L39
  constraint perpendicular L10 L40
  constraint perpendicular L10 L41
  constraint perpendicular L22 L42
  constraint perpendicular L22 L43
extrude "Extrude7" cut sketch "Sketch3" against normal blind 35 contours L4 S0 L36 L37 | S0 | L26 S0 L34 L35 | L16 S0 L38 L39 | L14 S0 L32 L33 | L10 S0 L40 L41 | L8 S0 L30 L31 | L22 S0 L42 L43 | L20 S0 L28 L29 picked at (28.622103, 33.890194) picked at (-3.487087, 5.211904) picked at (38.482385, 9.691279) picked at (-7.176077, 36.711758) picked at (32.073698, -27.223671) picked at (-34.764198, 30.927362) picked at (9.510854, -36.812994) picked at (-38.573884, -11.308492) picked at (-31.119988, -31.880788)
fillet "Fillet4" radius 1 16 edges at (-36.964405, 8.794291, 1.5) (-37.317874, 15.291931, 1.5) (-32.790801, 29.49158, 1.5) (-28.770264, 30.348131, 1.5) (12.116839, 35.729853, 1.5) (7.610633, 34.938941, 1.5) (25.919241, 29.71354, 1.5) (26.175138, 26.186531, 1.5) (36.68528, -17.009632, 1.5) (35.421022, -11.561507, 1.5) (27.102043, -32.066301, 1.5) (31.281435, -29.423422, 1.5) (-6.519453, -35.341542, 1.5) (-9.625144, -38.169628, 1.5) (-32.415986, -34.172982, 1.5) (-33.002634, -29.537862, 1.5)
other "Sketch1 (2)"
extrude "Extrude9" cut sketch "sketch 2514" along normal blind 11 contours A34 | A35 | A36 | A37 picked at (14.32473, -46.566988) picked at (-47.372111, -13.734435) picked at (46.62789, 14.265565) picked at (-14.111261, 47.487465)
sketch "Sketch4" plane through (0, 0, 3) normal (0, 0, 1) x (-1, 0, 0)
  spline S0 degree 3 poles (33.028609, 28.071836) (33.020542, 28.201801) (33.037938, 28.332099) (33.121694, 28.578692) (33.187255, 28.69263) (33.35836, 28.888963) (33.462269, 28.969481) (33.695102, 29.086154) (33.821799, 29.121194) (34.01862, 29.136006) (34.085931, 29.134286) (34.219188, 29.117378) (34.284796, 29.102233) (34.348388, 29.080627) knots 0 0 0 0 0.03906445 0.03906445 0.07812889 0.07812889 0.11719334 0.11719334 0.15625779 0.15625779 0.17640658 0.17640658 0.19655538 0.19655538 0.19655538 0.19655538
  spline S1 degree 3 poles (33.028609, 28.071836) (33.070325, 27.399743) (33.167612, 26.697689) (33.534795, 25.632572) (33.720748, 25.326789) (34.102443, 24.870238) (34.323648, 24.704363) (34.841834, 24.437201) (35.152732, 24.346965) (36.444281, 24.071142) (37.766512, 23.970732) (40.258569, 22.861355) (41.159058, 22.248794) (42.580431, 20.763821) (43.105542, 19.944649) (43.820617, 18.088798) (43.981774, 17.098841) (44.002724, 14.699008) (43.726283, 13.299817) (42.523118, 9.293833) (41.144668, 6.638018) (39.093015, 2.019583) (38.33328, 0.102917) (37.445131, -3.451458) (37.219765, -4.824183) (37.092807, -6.21584) knots 0.12920252 0.12920252 0.12920252 0.12920252 0.29400635 0.29400635 0.41743504 0.41743504 0.55008159 0.55008159 0.70447822 0.70447822 1.12919382 1.12919382 1.40886872 1.40886872 1.66213987 1.66213987 1.92272299 1.92272299 2.28120027 2.28120027 3.00174739 3.00174739 3.49260172 3.49260172 3.80923678 3.80923678 3.80923678 3.80923678
  spline S2 degree 3 poles (38.088834, -7.30669) (37.958619, -7.306711) (37.829645, -7.281298) (37.588698, -7.182465) (37.479028, -7.10999) (37.293642, -6.927081) (37.219699, -6.818395) (37.13638, -6.622803) (37.113583, -6.543309) (37.088005, -6.380538) (37.085323, -6.297883) (37.092807, -6.21584) knots 0 0 0 0 0.03906445 0.03906445 0.07812889 0.07812889 0.11719334 0.11719334 0.14190861 0.14190861 0.16662387 0.16662387 0.16662387 0.16662387
  line L0 (38.088834, -7.30669) -> (44.477012, 2.623123)
  arc A0 (49.249836, -0.9845) -> (44.477012, 2.623123) centre (47.000001, 1) ccw
  line L1 (49.249836, -0.9845) -> (41.439374, -9.839254)
  line L2 (41.439374, -9.839254) -> (37.553028, -14.980826)
  spline S3 degree 3 poles (37.355491, -15.680812) (37.343423, -15.556976) (37.354571, -15.431969) (37.422156, -15.192477) (37.478002, -15.080084) (37.553028, -14.980826) knots 0 0 0 0 0.03732672 0.03732672 0.07465345 0.07465345 0.07465345 0.07465345
  spline S4 degree 3 poles (37.355491, -15.680812) (37.717512, -19.395606) (38.115975, -22.808309) (37.32032, -26.055888) (37.037048, -26.721878) (36.287107, -27.771965) (35.864089, -28.165019) (34.777138, -28.862662) (34.111926, -29.125105) (33.399815, -29.330821) knots 0.03917141 0.03917141 0.03917141 0.03917141 1.16482767 1.16482767 1.51694644 1.51694644 1.81940977 1.81940977 2.17139083 2.17139083 2.17139083 2.17139083
  spline S5 degree 3 poles (32.689476, -30.136274) (32.709693, -30.007638) (32.754843, -29.884181) (32.889924, -29.661523) (32.978563, -29.56445) (33.178711, -29.416652) (33.285884, -29.363733) (33.399815, -29.330821) knots 0 0 0 0 0.03906445 0.03906445 0.07812889 0.07812889 0.11370578 0.11370578 0.11370578 0.11370578
  line L3 (32.689476, -30.136274) -> (31.798898, -35.802654)
  line L4 (31.798898, -35.802654) -> (29.963534, -47.466334)
  arc A1 (24.140467, -46.09277) -> (29.963534, -47.466334) centre (27, -47.000001) ccw
  line L5 (24.140467, -46.09277) -> (27.711083, -34.838407)
  line L6 (27.711083, -34.838407) -> (28.342134, -32.16314)
  spline S6 degree 3 poles (26.916548, -31.04169) (27.032682, -30.982795) (27.15921, -30.947146) (27.418808, -30.926354) (27.549397, -30.94141) (27.797453, -31.020732) (27.912548, -31.084239) (28.111917, -31.251796) (28.194285, -31.354245) (28.310066, -31.575309) (28.346065, -31.690083) (28.375918, -31.926876) (28.369531, -32.046994) (28.342134, -32.16314) knots 0 0 0 0 0.03906445 0.03906445 0.07812889 0.07812889 0.11719334 0.11719334 0.15625779 0.15625779 0.1920579 0.1920579 0.227858 0.227858 0.227858 0.227858
  spline S7 degree 3 poles (26.916548, -31.04169) (26.501678, -31.252085) (26.107211, -31.499509) (24.939768, -32.410184) (24.29803, -33.165919) (22.091994, -36.254574) (20.565282, -39.28296) (15.831093, -43.406948) (14.024745, -44.411258) (11.181859, -45.397232) (9.989834, -45.607) (8.140393, -45.536834) (7.398883, -45.389219) (6.139798, -44.814776) (5.640001, -44.453149) (4.7208, -43.481488) (4.349579, -42.883055) (3.462916, -41.050115) (3.101277, -39.69498) (2.31369, -37.647221) (1.945545, -36.882494) (1.036613, -35.79784) (0.593737, -35.439307) (-0.469029, -34.890024) (-1.078331, -34.709667) (-2.902765, -34.442063) (-4.21808, -34.494421) (-5.659673, -34.662249) knots 0.20837114 0.20837114 0.20837114 0.20837114 0.35937386 0.35937386 0.67047774 0.67047774 1.4465987 1.4465987 1.89541729 1.89541729 2.22492207 2.22492207 2.45047306 2.45047306 2.6397202 2.6397202 2.85015814 2.85015814 3.24794097 3.24794097 3.51947787 3.51947787 3.71561689 3.71561689 3.91564309 3.91564309 4.24291454 4.24291454 4.24291454 4.24291454
  spline S8 degree 3 poles (-6.267359, -36.346049) (-6.357274, -36.251862) (-6.427932, -36.141013) (-6.52278, -35.898469) (-6.546064, -35.769094) (-6.54173, -35.5087) (-6.514153, -35.380172) (-6.411285, -35.140919) (-6.336977, -35.032483) (-6.165307, -34.864241) (-6.074436, -34.800666) (-5.875645, -34.705715) (-5.769085, -34.674986) (-5.659673, -34.662249) knots 0 0 0 0 0.03906445 0.03906445 0.07812889 0.07812889 0.11719334 0.11719334 0.15625779 0.15625779 0.18930324 0.18930324 0.2223487 0.2223487 0.2223487 0.2223487
  line L7 (-6.267359, -36.346049) -> (-5.767132, -36.870049)
  line L8 (-5.767132, -36.870049) -> (3.007378, -44.770554)
  arc A2 (-1.320176, -48.901784) -> (3.007378, -44.770554) centre (1, -47.000001) ccw
  line L9 (-1.320176, -48.901784) -> (-11.749599, -36.177887)
  spline S9 degree 3 poles (-12.684916, -35.825011) (-12.55642, -35.803926) (-12.425033, -35.808141) (-12.191152, -35.862108) (-12.088945, -35.904256) (-11.902341, -36.020074) (-11.819212, -36.092959) (-11.749599, -36.177887) knots 0 0 0 0 0.03906445 0.03906445 0.07200812 0.07200812 0.1049518 0.1049518 0.1049518 0.1049518
  spline S10 degree 3 poles (-12.684916, -35.825011) (-15.152305, -36.229886) (-17.56612, -36.507138) (-20.617728, -36.140773) (-21.595405, -35.894944) (-23.151598, -35.065944) (-23.73315, -34.591978) (-24.687849, -33.42352) (-25.03938, -32.77321) (-25.502185, -31.577004) (-25.653053, -31.047073) (-25.769625, -30.511953) knots 0.05769777 0.05769777 0.05769777 0.05769777 0.81058803 0.81058803 1.16886844 1.16886844 1.44619299 1.44619299 1.71282967 1.71282967 1.90895598 1.90895598 1.90895598 1.90895598
  spline S11 degree 3 poles (-26.760211, -29.724895) (-26.630008, -29.723137) (-26.500707, -29.746827) (-26.258463, -29.842438) (-26.147836, -29.913444) (-25.982773, -30.072013) (-25.922122, -30.150529) (-25.825786, -30.322765) (-25.790628, -30.41554) (-25.769625, -30.511953) knots 0 0 0 0 0.03906445 0.03906445 0.07812889 0.07812889 0.107731 0.107731 0.13733311 0.13733311 0.13733311 0.13733311
  line L10 (-26.760211, -29.724895) -> (-35.15287, -29.83822)
  line L11 (-35.15287, -29.83822) -> (-46.958966, -29.99972)
  arc A3 (-46.588905, -24.0283) -> (-46.958966, -29.99972) centre (-47.000001, -27) ccw
  line L12 (-46.588905, -24.0283) -> (-34.893086, -25.646262)
  line L13 (-34.893086, -25.646262) -> (-27.2325, -26.121004)
  spline S12 degree 3 poles (-26.170767, -25.138463) (-26.172791, -25.268662) (-26.200227, -25.397221) (-26.302832, -25.636586) (-26.377021, -25.745104) (-26.562819, -25.927594) (-26.672653, -25.999821) (-26.862592, -26.077231) (-26.934903, -26.097616) (-27.082715, -26.121857) (-27.15775, -26.125636) (-27.2325, -26.121004) knots 0 0 0 0 0.03906445 0.03906445 0.07812889 0.07812889 0.11719334 0.11719334 0.13966134 0.13966134 0.16212934 0.16212934 0.16212934 0.16212934
  spline S13 degree 3 poles (-26.170767, -25.138463) (-26.10385, -20.833987) (-25.471174, -16.204979) (-26.544717, -7.681658) (-27.73616, -4.599407) (-31.188004, 2.436605) (-33.265635, 6.07333) (-34.771789, 9.827038) knots 0.10413309 0.10413309 0.10413309 0.10413309 1.3791009 1.3791009 2.41617104 2.41617104 3.40624296 3.40624296 3.40624296 3.40624296
  spline S14 degree 3 poles (-36.512881, 10.036897) (-36.437064, 10.142763) (-36.341294, 10.232809) (-36.120628, 10.371122) (-35.997843, 10.418066) (-35.741188, 10.462248) (-35.609773, 10.459062) (-35.35556, 10.402497) (-35.235194, 10.349658) (-35.048762, 10.219811) (-34.977667, 10.153102) (-34.856917, 10.001316) (-34.807902, 9.917042) (-34.771789, 9.827038) knots 0 0 0 0 0.03906445 0.03906445 0.07812889 0.07812889 0.11719334 0.11719334 0.15625779 0.15625779 0.18535143 0.18535143 0.21444508 0.21444508 0.21444508 0.21444508
  line L14 (-36.512881, 10.036897) -> (-38.305738, 7.533451)
  line L15 (-38.305738, 7.533451) -> (-44.436043, -2.557602)
  arc A4 (-49.300203, 0.925894) -> (-44.436043, -2.557602) centre (-47.000001, -1) ccw
  line L16 (-49.300203, 0.925894) -> (-41.720395, 9.978878)
  line L17 (-41.720395, 9.978878) -> (-36.901029, 16.708373)
  spline S15 degree 3 poles (-36.717088, 17.368596) (-36.707973, 17.252065) (-36.71936, 17.134833) (-36.782101, 16.909635) (-36.832972, 16.803404) (-36.901029, 16.708373) knots 0 0 0 0 0.03506615 0.03506615 0.07013231 0.07013231 0.07013231 0.07013231
  spline S16 degree 3 poles (-36.717088, 17.368596) (-36.851793, 19.090796) (-36.725294, 20.800665) (-35.82491, 23.830023) (-35.192711, 25.085877) (-33.574997, 27.33099) (-32.636218, 28.298843) (-31.606983, 29.157724) knots 0.03608701 0.03608701 0.03608701 0.03608701 0.555731 0.555731 0.98365139 0.98365139 1.38609526 1.38609526 1.38609526 1.38609526
  spline S17 degree 3 poles (-31.250302, 29.853272) (-31.259708, 29.723397) (-31.294392, 29.596602) (-31.383142, 29.418243) (-31.420195, 29.359812) (-31.50574, 29.251513) (-31.554002, 29.201936) (-31.606983, 29.157724) knots 0 0 0 0 0.03906445 0.03906445 0.05976579 0.05976579 0.08046713 0.08046713 0.08046713 0.08046713
  line L18 (-31.250302, 29.853272) -> (-30.845628, 35.440539)
  line L19 (-30.845628, 35.440539) -> (-29.992153, 47.216854)
  arc A5 (-24.074611, 46.335098) -> (-29.992153, 47.216854) centre (-27, 47.000001) ccw
  line L20 (-24.074611, 46.335098) -> (-26.691493, 34.821543)
  line L21 (-26.691493, 34.821543) -> (-26.827892, 33.906158)
  spline S18 degree 3 poles (-25.443022, 32.840437) (-25.562603, 32.788899) (-25.691108, 32.761211) (-25.951498, 32.756651) (-26.080893, 32.779823) (-26.323519, 32.874462) (-26.434429, 32.945024) (-26.62296, 33.12469) (-26.698777, 33.232076) (-26.790548, 33.437548) (-26.816707, 33.529187) (-26.842431, 33.717075) (-26.841866, 33.812373) (-26.827892, 33.906158) knots 0 0 0 0 0.03906445 0.03906445 0.07812889 0.07812889 0.11719334 0.11719334 0.15625779 0.15625779 0.1847039 0.1847039 0.21315002 0.21315002 0.21315002 0.21315002
  spline S19 degree 3 poles (-25.443022, 32.840437) (-22.639111, 34.048877) (-19.64058, 34.864689) (-13.990802, 35.609538) (-11.903288, 35.347809) (-8.639296, 34.492873) (-7.24095, 33.736993) (-4.677922, 32.21498) (-3.539006, 31.471178) (-1.766627, 30.825805) (-1.13553, 30.690347) (0.120331, 30.722159) (0.684409, 30.86072) (1.959514, 31.399025) (2.667406, 31.871418) (4.176502, 33.086706) (4.982409, 33.852701) (5.832592, 34.675606) knots 0.18219729 0.18219729 0.18219729 0.18219729 1.09067944 1.09067944 2.11663156 2.11663156 3.31549349 3.31549349 4.45967423 4.45967423 5.07162521 5.07162521 5.62607132 5.62607132 6.35980303 6.35980303 7.15795757 7.15795757 7.15795757 7.15795757
  spline S20 degree 3 poles (5.885742, 36.057127) (5.972072, 35.959644) (6.038536, 35.84623) (6.124249, 35.600309) (6.142679, 35.470154) (6.128612, 35.210105) (6.096249, 35.082697) (5.989005, 34.856928) (5.918623, 34.758878) (5.832592, 34.675606) knots 0 0 0 0 0.03906445 0.03906445 0.07812889 0.07812889 0.11719334 0.11719334 0.15311273 0.15311273 0.15311273 0.15311273
  line L22 (5.885742, 36.057127) -> (5.383635, 36.624105)
  line L23 (5.383635, 36.624105) -> (-3.089335, 44.84717)
  arc A6 (1.389663, 48.813702) -> (-3.089335, 44.84717) centre (-1, 47.000001) ccw
  line L24 (1.389663, 48.813702) -> (8.527907, 39.408625)
  line L25 (8.527907, 39.408625) -> (8.997232, 38.878665)
  spline S21 degree 3 poles (10.353438, 38.74738) (10.250013, 38.668265) (10.132124, 38.610108) (9.880688, 38.542257) (9.749546, 38.53321) (9.500962, 38.564658) (9.385265, 38.601194) (9.172426, 38.713607) (9.077022, 38.788566) (8.997232, 38.878665) knots 0 0 0 0 0.03906445 0.03906445 0.07812889 0.07812889 0.11423407 0.11423407 0.15033925 0.15033925 0.15033925 0.15033925
  spline S22 degree 3 poles (10.353438, 38.74738) (11.733539, 39.803082) (13.210331, 40.705104) (16.432276, 41.90028) (18.061322, 42.165253) (21.42658, 42.026481) (23.073064, 41.629511) (26.565289, 40.202857) (28.314525, 39.054702) (30.298495, 37.237861) (30.878286, 36.616261) (31.702413, 35.507726) (32.000821, 35.03614) (32.246808, 34.538749) knots 0.09311255 0.09311255 0.09311255 0.09311255 0.61605828 0.61605828 1.12703458 1.12703458 1.63347766 1.63347766 2.26940705 2.26940705 2.55315447 2.55315447 2.74216348 2.74216348 2.74216348 2.74216348
  spline S23 degree 3 poles (32.821479, 34.035211) (32.698186, 34.077101) (32.584254, 34.142673) (32.38663, 34.314936) (32.305301, 34.420473) (32.246808, 34.538749) knots 0 0 0 0 0.03906445 0.03906445 0.07864923 0.07864923 0.07864923 0.07864923
  line L26 (32.821479, 34.035211) -> (36.313471, 32.848768)
  line L27 (36.313471, 32.848768) -> (47.747888, 29.90528)
  arc A7 (45.823197, 24.240447) -> (47.747889, 29.905282) centre (47.000001, 27) ccw
  line L28 (45.823197, 24.240447) -> (34.962331, 28.872033)
  line L29 (34.962331, 28.872033) -> (34.348388, 29.080627)
  arc A8 (55, 15) -> (15, 55) centre (15, 15) ccw
  line L30 (15, 55) -> (-15, 55)
  arc A9 (-15, 55) -> (-55, 15) centre (-15, 15) ccw
  line L31 (-55, 15) -> (-55, -15)
  arc A10 (-55, -15) -> (-15, -55) centre (-15, -15) ccw
  line L32 (-15, -55) -> (15, -55)
  arc A11 (15, -55) -> (55, -15) centre (15, -15) ccw
  line L33 (55, -15) -> (55, 15)
  circle A12 centre (-14, 47.000001) radius 1.5
  circle A13 centre (47.000001, 14) radius 1.5
  circle A14 centre (-47.000001, -14) radius 1.5
  circle A15 centre (14, -47.000001) radius 1.5
  circle A16 centre (47.000001, -22) radius 1.5
  circle A17 centre (-21.042031, -45.95674) radius 1.5
  circle A18 centre (19.806368, 49.24591) radius 1.5
  circle A19 centre (-47.207036, 20.58349) radius 1.5
  circle A20 centre (-38.15, -37.75) radius 1.25
  circle A21 centre (37.75, -38.15) radius 1.25
  circle A22 centre (38.15, 37.75) radius 1.25
  circle A23 centre (-37.75, 38.15) radius 1.25
  circle A24 centre (-38.15, -37.75) radius 2.75
  circle A25 centre (-37.75, 38.15) radius 2.75
  circle A26 centre (38.15, 37.75) radius 2.75
  circle A27 centre (37.75, -38.15) radius 2.75
  dimension "d123" = 3
  dimension "d124" = 3
  dimension "d125" = 3
  dimension "d126" = 3
  dimension "d129" = 5.5
  dimension "d130" = 5.5
  dimension "d131" = 5.5
  dimension "d132" = 5.5
  constraint concentric A20 A24
  constraint concentric A23 A25
  constraint concentric A22 A26
  constraint concentric A21 A27
  measures "d123" diameter of A16
  measures "d124" diameter of A17
  measures "d125" diameter of A18
  measures "d126" diameter of A19
  measures "d129" diameter of A24
  measures "d130" diameter of A25
  measures "d131" diameter of A26
  measures "d132" diameter of A27
extrude "Extrude10" cut sketch "Sketch4" against normal blind 20 contours A16 | A17 | A18 | A19 picked at (47.410458, -21.517493) picked at (-21.766895, -46.281368) picked at (19.061952, 49.050995) picked at (-46.796579, 21.065997)
extrude "Extrude11" cut sketch "Sketch4" against normal blind 30 contours A20 | A21 | A22 | A23 | A24 | A25 | A26 | A27 picked at (-39.030134, -37.847182) picked at (36.869866, -38.247182) picked at (37.269866, 37.652818) picked at (-38.630134, 38.052818) picked at (-35.914892, -37.948723) picked at (-35.514892, 37.951277) picked at (40.385108, 37.551277) picked at (39.985108, -38.348723)